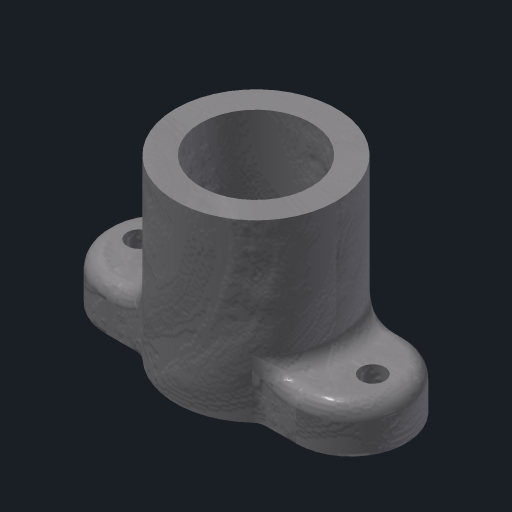
# Autodesk Inventor part: ACOPLE_LINEAL
Saved by Autodesk Inventor 2024.3 (Build 283343000, 343)
## iProperties
Created: 2024-06-26
Part Number: ACOPLE_LINEAL
Material: Steel, Mild, Welded
Document SubType Name: Modeling
Designer: Niler
Density: 7.85 g/cm^3
Appearance: Weld - Steel Mild
Author: Niler
Autodesk Inventor part; units mm, degrees
ref_plane "YZ Plane" through (0, 0, 0) normal (1, 0, 0) x (0, 1, 0)
ref_plane "XZ Plane" through (0, 0, 0) normal (0, 1, 0) x (-1, 0, 0)
ref_plane "XY Plane" through (0, 0, 0) normal (0, 0, 1) x (1, 0, 0)
sketch "Sketch1" plane through (0, 0, 0) normal (0, 1, 0) x (-1, 0, 0)
  circle A0 centre (0, 0) radius 11
  circle A1 centre (0, 0) radius 7.575
  dimension "d0" = 22
  dimension "d1" = 15.15
  constraints: 2 centre point, 2 coincident
  measures "d0" diameter of A0
  measures "d1" diameter of A1
extrude "Extrusion1" add sketch "Sketch1" along normal blind 24
sketch "Sketch2" plane through (0, 0, 0) normal (0, -1, 0) x (1, 0, 0)
  circle A0 centre (0, 0) radius 11 projected
  circle A1 centre (0, 0) radius 7.575 projected
  line L0 (13, 0) -> (-13, 0) construction
  line L1 (13, 7.5) -> (-13, 7.5)
  line L2 (-13, -7.5) -> (13, -7.5)
  arc A2 (13, -7.5) -> (13, 7.5) centre (13, 0) ccw
  arc A3 (-13, 7.5) -> (-13, -7.5) centre (-13, 0) ccw
  circle A4 centre (-16, 0) radius 1.65
  line L3 (0, 0) -> (0, -4.5395) construction
  circle A5 centre (16, 0) radius 1.65
  point P0 (-8.0467, -7.5)
  point P1 (-8.0467, 7.5)
  point P2 (8.0467, 7.5)
  point P3 (8.0467, -7.5)
  dimension "d4" = 15
  dimension "d5" = 26
  dimension "d7" = 3.3
  dimension "d8" = 16
  constraints: 10 end point, 4 centre point, 4 point on circle, 4 tangent, 1 horizontal, 1 horizontal alignment, 1 midpoint, 1 parallel, 1 symmetric about line, 1 vertical, 1 other
  measures "d4" distance between parallel lines of L1 L2
  measures "d5" distance of L0.end L0.start
  measures "d7" diameter of A4
  measures "d8" distance from line of L3 A4.centre
extrude "Extrusion2" add sketch "Sketch2" against normal blind 6 contours A0 L1 A2 L2 | A0 L2 A3 L1
fillet "Fillet1" radius 2 3 edges at (11, 6, 0) (-10.2351, 6, 4.0303) (-10.2351, 6, -4.0303)
fillet "Fillet2" radius 2 8 edges at (-8.0467, 7, -7.5) (-8.0467, 3, -7.5) (8.0467, 3, -7.5) (8.0467, 7, -7.5) (8.0467, 3, 7.5) (8.0467, 7, 7.5) (-8.0467, 7, 7.5) (-8.0467, 3, 7.5)
fillet "Fillet3" radius 2 16 edges at (-11.8092, 6, 7.5) (-9.7013, 6.141, 7.5) (-8.1046, 7.2461, 7.654) (-11.8092, 6, -7.5) (-9.7013, 6.141, -7.5) (-8.509, 6.8485, -7.5336) (-7.8187, 7.5786, -7.8012) (-20.5, 6, 0) (11.8092, 6, -7.5) (9.7013, 6.141, -7.5) (8.1045, 7.2461, -7.654) (11.8092, 6, 7.5) (9.7013, 6.141, 7.5) (7.8187, 7.5786, 7.8012) (8.509, 6.8485, 7.5336) (20.5, 6, 0)
body "Solid1"
